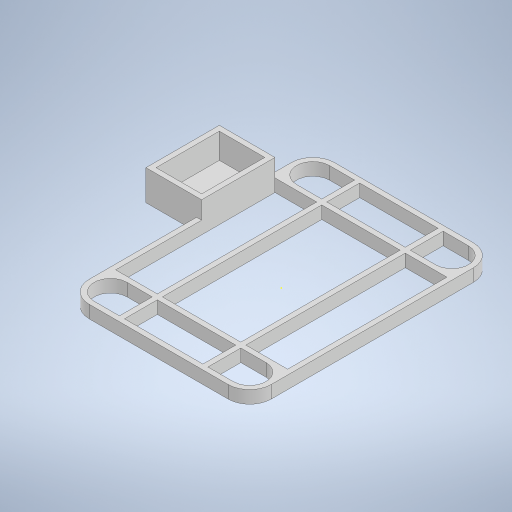
# Autodesk Inventor part: Stand Brace
Saved by Autodesk Inventor 2024.1 (Build 281209000, 209)
## iProperties
Created: 2024-01-03
Part Number: Stand Brace
Material: Generic
Document SubType Name: Modeling
Designer: ryanm
Density: 1 g/cm^3
Appearance: Default
Author: ryanm
Autodesk Inventor part; units mm, degrees
ref_plane "YZ Plane" through (0, 0, 0) normal (1, 0, 0) x (0, 1, 0)
ref_plane "XZ Plane" through (0, 0, 0) normal (0, 1, 0) x (-1, 0, 0)
ref_plane "XY Plane" through (0, 0, 0) normal (0, 0, 1) x (1, 0, 0)
sketch "Sketch1" plane through (0, 0, 0) normal (0, 1, 0) x (-1, 0, 0)
  line L0 (36, 40) -> (36, 0)
  arc A0 (36, 40) -> (27.5, 48.5) centre (27.5, 40) ccw
  line L1 (27.5, 48.5) -> (0, 48.5)
  line L2 (0, 48.5) -> (0, 0) construction
  arc A1 (27.5, 33.5) -> (27.5, 46.5) centre (27.5, 40) ccw
  line L3 (27.5, 46.5) -> (17.5, 46.5)
  line L4 (17.5, 33.5) -> (27.5, 33.5)
  line L5 (17.5, 33.5) -> (17.5, 46.5)
  line L6 (17.5, 31.5) -> (17.5, 0)
  line L7 (15.5, 33.5) -> (0, 33.5)
  line L8 (15.5, 46.5) -> (0, 46.5)
  line L9 (15.5, 46.5) -> (15.5, 33.5)
  line L10 (15.5, 31.5) -> (15.5, 0)
  line L11 (34, 31.5) -> (17.5, 31.5)
  line L12 (15.5, 31.5) -> (0, 31.5)
  line L13 (34, 31.5) -> (34, 0)
  line L14 (36, 0) -> (0, 0) construction
  line L15 (-36, 40) -> (-36, 0)
  line L16 (-27.5, 48.5) -> (0, 48.5)
  arc A2 (-27.5, 48.5) -> (-36, 40) centre (-27.5, 40) ccw
  arc A3 (-27.5, 46.5) -> (-27.5, 33.5) centre (-27.5, 40) ccw
  line L17 (-27.5, 46.5) -> (-17.5, 46.5)
  line L18 (-17.5, 33.5) -> (-27.5, 33.5)
  line L19 (-17.5, 33.5) -> (-17.5, 46.5)
  line L20 (-17.5, 31.5) -> (-17.5, 0)
  line L21 (-15.5, 33.5) -> (0, 33.5)
  line L22 (-15.5, 46.5) -> (0, 46.5)
  line L23 (-15.5, 46.5) -> (-15.5, 33.5)
  line L24 (-15.5, 31.5) -> (-15.5, 0)
  line L25 (-34, 31.5) -> (-17.5, 31.5)
  line L26 (-15.5, 31.5) -> (0, 31.5)
  line L27 (-34, 31.5) -> (-34, 0)
  line L28 (36, -40) -> (36, 0)
  line L29 (27.5, -48.5) -> (0, -48.5)
  arc A4 (27.5, -48.5) -> (36, -40) centre (27.5, -40) ccw
  line L30 (0, -48.5) -> (0, 0) construction
  arc A5 (27.5, -46.5) -> (27.5, -33.5) centre (27.5, -40) ccw
  line L31 (27.5, -46.5) -> (17.5, -46.5)
  line L32 (17.5, -33.5) -> (27.5, -33.5)
  line L33 (17.5, -33.5) -> (17.5, -46.5)
  line L34 (17.5, -31.5) -> (17.5, 0)
  line L35 (15.5, -33.5) -> (0, -33.5)
  line L36 (15.5, -46.5) -> (0, -46.5)
  line L37 (15.5, -46.5) -> (15.5, -33.5)
  line L38 (15.5, -31.5) -> (15.5, 0)
  line L39 (34, -31.5) -> (17.5, -31.5)
  line L40 (15.5, -31.5) -> (0, -31.5)
  line L41 (34, -31.5) -> (34, 0)
  line L42 (-36, -40) -> (-36, 0)
  line L43 (-17.5, -31.5) -> (-17.5, 0)
  line L44 (-15.5, -31.5) -> (-15.5, 0)
  line L45 (-34, -31.5) -> (-34, 0)
  line L46 (-34, -31.5) -> (-17.5, -31.5)
  line L47 (-17.5, -33.5) -> (-27.5, -33.5)
  arc A6 (-27.5, -33.5) -> (-27.5, -46.5) centre (-27.5, -40) ccw
  arc A7 (-36, -40) -> (-27.5, -48.5) centre (-27.5, -40) ccw
  line L48 (-15.5, -31.5) -> (0, -31.5)
  line L49 (-15.5, -33.5) -> (0, -33.5)
  line L50 (-17.5, -33.5) -> (-17.5, -46.5)
  line L51 (-15.5, -46.5) -> (-15.5, -33.5)
  line L52 (-27.5, -48.5) -> (0, -48.5)
  line L53 (-27.5, -46.5) -> (-17.5, -46.5)
  line L54 (-15.5, -46.5) -> (0, -46.5)
  point P0 (34, 40)
  point P1 (-34, 40)
  point P2 (34, -40)
  point P3 (-34, -40)
  dimension "d42" = 13
  dimension "d43" = 10
  dimension "d45" = 2
  dimension "d46" = 2
  dimension "d47" = 48.5
  dimension "d48" = 27.5
  dimension "d49" = 2
  dimension "d50" = 2
  dimension "d51" = 2
  dimension "d53" = 31.5
  constraints: 110 end point, 51 symmetric about line, 17 point on circle, 8 centre point, 8 point on line, 6 coincident, 6 horizontal alignment, 5 perpendicular, 5 vertical alignment, 4 vertical, 3 tangent, 2 horizontal, 1 parallel, 6 other
  measures "d42" diameter of A1
  measures "d43" distance of L3.start L3.end
  measures "d45" distance between parallel lines of L1 L3
  measures "d46" distance from line of L0 point (34, 40)
  measures "d47" distance of L2.start L2.end
  measures "d48" distance from line of L2 A0.centre
  measures "d49" distance between parallel lines of L9 L5
  measures "d50" distance between parallel lines of L11 L4
  measures "d51" distance between parallel lines of L0 L13
  measures "d53" distance from line of L13.end L11
extrude "Extrusion1" add sketch "Sketch1" along normal blind 5
sketch "Sketch4" plane through (0, 0, 0) normal (0, -1, 0) x (1, 0, 0)
  point P0 (0, 0)
sketch "Sketch5" plane through (0, 0, 0) normal (0, 1, 0) x (-1, 0, 0)
  line L0 (27.5, 48.5) -> (-27.5, 48.5) projected
  arc A0 (-27.5, 48.5) -> (-36, 40) centre (-27.5, 40) ccw projected
  line L1 (-36, 40) -> (-36, -40) projected
  arc A1 (-36, -40) -> (-27.5, -48.5) centre (-27.5, -40) ccw projected
  line L2 (-27.5, -48.5) -> (27.5, -48.5) projected
  arc A2 (27.5, -48.5) -> (36, -40) centre (27.5, -40) ccw projected
  line L3 (36, -40) -> (36, 40) projected
  arc A3 (36, 40) -> (27.5, 48.5) centre (27.5, 40) ccw projected
  line L4 (-17.5, -33.5) -> (-17.5, -46.5) projected
  line L5 (-17.5, -46.5) -> (-27.5, -46.5) projected
  arc A4 (-27.5, -33.5) -> (-27.5, -46.5) centre (-27.5, -40) ccw projected
  line L6 (-27.5, -33.5) -> (-17.5, -33.5) projected
  line L7 (-15.5, -46.5) -> (-15.5, -33.5) projected
  line L8 (-15.5, -33.5) -> (15.5, -33.5) projected
  line L9 (15.5, -33.5) -> (15.5, -46.5) projected
  line L10 (15.5, -46.5) -> (-15.5, -46.5) projected
  line L11 (27.5, -46.5) -> (17.5, -46.5) projected
  line L12 (17.5, -46.5) -> (17.5, -33.5) projected
  line L13 (17.5, -33.5) -> (27.5, -33.5) projected
  arc A5 (27.5, -46.5) -> (27.5, -33.5) centre (27.5, -40) ccw projected
  line L14 (-27.5, 46.5) -> (-17.5, 46.5) projected
  line L15 (-17.5, 46.5) -> (-17.5, 33.5) projected
  line L16 (-17.5, 33.5) -> (-27.5, 33.5) projected
  arc A6 (-27.5, 46.5) -> (-27.5, 33.5) centre (-27.5, 40) ccw projected
  line L17 (-34, 31.5) -> (-17.5, 31.5) projected
  line L18 (-17.5, 31.5) -> (-17.5, -31.5) projected
  line L19 (-17.5, -31.5) -> (-34, -31.5) projected
  line L20 (-34, -31.5) -> (-34, 31.5) projected
  line L21 (-15.5, 31.5) -> (15.5, 31.5) projected
  line L22 (15.5, 31.5) -> (15.5, -31.5) projected
  line L23 (15.5, -31.5) -> (-15.5, -31.5) projected
  line L24 (-15.5, -31.5) -> (-15.5, 31.5) projected
  line L25 (15.5, 46.5) -> (15.5, 33.5) projected
  line L26 (15.5, 33.5) -> (-15.5, 33.5) projected
  line L27 (-15.5, 33.5) -> (-15.5, 46.5) projected
  line L28 (-15.5, 46.5) -> (15.5, 46.5) projected
  line L29 (34, 31.5) -> (34, -31.5) projected
  line L30 (34, -31.5) -> (17.5, -31.5) projected
  line L31 (17.5, -31.5) -> (17.5, 31.5) projected
  line L32 (17.5, 31.5) -> (34, 31.5) projected
  line L33 (17.5, 33.5) -> (17.5, 46.5) projected
  line L34 (17.5, 46.5) -> (27.5, 46.5) projected
  arc A7 (27.5, 33.5) -> (27.5, 46.5) centre (27.5, 40) ccw projected
  line L35 (27.5, 33.5) -> (17.5, 33.5) projected
  line L36 (36, -31.5) -> (56, -31.5)
  line L37 (56, -31.5) -> (56, -2.5)
  line L38 (56, -2.5) -> (36, -2.5)
  point P0 (0, 0)
  dimension "d54" = 20
  dimension "d55" = 29
  constraints: 6 end point, 2 perpendicular, 2 point on line, 1 horizontal, 1 horizontal alignment
  measures "d54" distance of L36.start L36.end
  measures "d55" distance of L36.end L37.end
extrude "Extrusion4" add sketch "Sketch5" along normal blind 2 contours L38 L37 L36 L3
sketch "Sketch6" plane through (0, 2, 0) normal (0, 1, 0) x (1, 0, 0)
  line L0 (-56, 2.5) -> (-36, 2.5) projected
  line L1 (-36, 31.5) -> (-36, 2.5) projected
  line L2 (-36, 31.5) -> (-56, 31.5) projected
  line L3 (-56, 31.5) -> (-56, 2.5) projected
  line L4 (-54, 29.5) -> (-36, 29.5)
  line L5 (-36, 4.5) -> (-54, 4.5)
  line L6 (-54, 4.5) -> (-54, 29.5)
  point P0 (0, 0)
  point P1 (-46, 2.5)
  dimension "d58" = 2
  dimension "d60" = 2
  constraints: 6 end point, 2 point on line, 2 vertical alignment, 1 midpoint, 1 perpendicular, 1 other
  measures "d58" distance between parallel lines of L2 L4
  measures "d60" distance from line of point (-46, 2.5) L5
extrude "Extrusion5" add sketch "Sketch6" along normal blind 10 contours L3 L2 L1 L4 L6 L5 L0
sketch "Sketch7" plane through (0, 5, 0) normal (0, 1, 0) x (1, 0, 0)
  line L0 (-36, 31.5) -> (-56, 31.5) projected
  line L1 (-34, -31.5) -> (-34, 31.5) projected
  line L2 (-36, 31.5) -> (-34, 31.5)
  line L3 (-36, 2.5) -> (-34, 2.5)
  line L4 (-27.5, -48.5) -> (27.5, -48.5) projected
  arc A0 (27.5, -48.5) -> (36, -40) centre (27.5, -40) ccw projected
  line L5 (36, -40) -> (36, 40) projected
  arc A1 (36, 40) -> (27.5, 48.5) centre (27.5, 40) ccw projected
  line L6 (27.5, 48.5) -> (-27.5, 48.5) projected
  arc A2 (-27.5, 48.5) -> (-36, 40) centre (-27.5, 40) ccw projected
  line L7 (-36, 40) -> (-36, 31.5) projected
  line L8 (-36, 31.5) -> (-36, 29.5) projected
  line L9 (-36, 29.5) -> (-36, 4.5) projected
  line L10 (-36, 4.5) -> (-36, 2.5) projected
  line L11 (-36, 2.5) -> (-36, -40) projected
  arc A3 (-36, -40) -> (-27.5, -48.5) centre (-27.5, -40) ccw projected
  line L12 (17.5, 33.5) -> (17.5, 46.5) projected
  line L13 (17.5, 46.5) -> (27.5, 46.5) projected
  arc A4 (27.5, 33.5) -> (27.5, 46.5) centre (27.5, 40) ccw projected
  line L14 (27.5, 33.5) -> (17.5, 33.5) projected
  line L15 (15.5, 46.5) -> (15.5, 33.5) projected
  line L16 (15.5, 33.5) -> (-15.5, 33.5) projected
  line L17 (-15.5, 33.5) -> (-15.5, 46.5) projected
  line L18 (-15.5, 46.5) -> (15.5, 46.5) projected
  line L19 (-27.5, 46.5) -> (-17.5, 46.5) projected
  line L20 (-17.5, 46.5) -> (-17.5, 33.5) projected
  line L21 (-17.5, 33.5) -> (-27.5, 33.5) projected
  arc A5 (-27.5, 46.5) -> (-27.5, 33.5) centre (-27.5, 40) ccw projected
  line L22 (27.5, -46.5) -> (17.5, -46.5) projected
  line L23 (17.5, -46.5) -> (17.5, -33.5) projected
  line L24 (17.5, -33.5) -> (27.5, -33.5) projected
  arc A6 (27.5, -46.5) -> (27.5, -33.5) centre (27.5, -40) ccw projected
  line L25 (34, -31.5) -> (17.5, -31.5) projected
  line L26 (17.5, -31.5) -> (17.5, 31.5) projected
  line L27 (17.5, 31.5) -> (34, 31.5) projected
  line L28 (34, 31.5) -> (34, -31.5) projected
  line L29 (15.5, -31.5) -> (-15.5, -31.5) projected
  line L30 (-15.5, -31.5) -> (-15.5, 31.5) projected
  line L31 (-15.5, 31.5) -> (15.5, 31.5) projected
  line L32 (15.5, 31.5) -> (15.5, -31.5) projected
  line L33 (-15.5, -46.5) -> (-15.5, -33.5) projected
  line L34 (-15.5, -33.5) -> (15.5, -33.5) projected
  line L35 (15.5, -33.5) -> (15.5, -46.5) projected
  line L36 (15.5, -46.5) -> (-15.5, -46.5) projected
  line L37 (-34, -31.5) -> (-34, 31.5) projected
  line L38 (-34, 31.5) -> (-17.5, 31.5) projected
  line L39 (-17.5, 31.5) -> (-17.5, -31.5) projected
  line L40 (-17.5, -31.5) -> (-34, -31.5) projected
  line L41 (-17.5, -33.5) -> (-17.5, -46.5) projected
  line L42 (-17.5, -46.5) -> (-27.5, -46.5) projected
  arc A7 (-27.5, -33.5) -> (-27.5, -46.5) centre (-27.5, -40) ccw projected
  line L43 (-27.5, -33.5) -> (-17.5, -33.5) projected
  point P0 (0, 0)
  constraints: 4 end point, 1 horizontal, 1 perpendicular, 1 point on line
extrude "Extrusion6" add sketch "Sketch7" along normal blind 7 contours L3 L10 L9 L8 L2 L1
equation "\"d50\" = d49"
equation "\"d51\" = d46"
equation "\"d60\" = d58"
equation "\"d21\" = d20"
equation "\"d33\" = d32"
equation "\"d20\" = 2"
equation "\"d32\" = 2"
body "Solid1"
